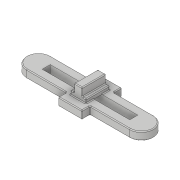
# Autodesk Inventor part: Slider1
Saved by Autodesk Inventor 2017 (Build 210142000, 142)
## iProperties
Created: 2016-07-28
Part Number: Slider1
Material: Generic
Document SubType Name: Modeling
Designer: Tutorial Books
Density: 1 g/cm^3
Appearance: Default
Author: Tutorial Books
Autodesk Inventor part; units mm, degrees
ref_plane "YZ Plane" through (0, 0, 0) normal (1, 0, 0) x (0, 1, 0)
ref_plane "XZ Plane" through (0, 0, 0) normal (0, 1, 0) x (-1, 0, 0)
ref_plane "XY Plane" through (0, 0, 0) normal (0, 0, 1) x (1, 0, 0)
sketch "Sketch1" plane through (0, 0, 0) normal (0, 1, 0) x (-1, 0, 0)
  arc A0 (64.897, -14.986) -> (64.897, 14.986) centre (64.897, 0) ccw
  arc A1 (-64.897, 14.986) -> (-64.897, -14.986) centre (-64.897, 0) ccw
  line L0 (64.897, 14.986) -> (14.986, 14.986)
  line L1 (14.986, 14.986) -> (14.986, 25.146)
  line L2 (14.986, 25.146) -> (-14.986, 25.146)
  line L3 (-14.986, 25.146) -> (-14.986, 14.986)
  line L4 (-14.986, 14.986) -> (-64.897, 14.986)
  line L5 (64.897, -14.986) -> (14.986, -14.986)
  line L6 (14.986, -14.986) -> (14.986, -25.146)
  line L7 (14.986, -25.146) -> (-14.986, -25.146)
  line L8 (-14.986, -25.146) -> (-14.986, -14.986)
  line L9 (-14.986, -14.986) -> (-64.897, -14.986)
  line L10 (0, 0) -> (0, -36.9179) construction
  line L11 (0, 0) -> (35.3103, 0) construction
  line L12 (55.245, 5.08) -> (-55.245, 5.08)
  line L13 (-55.245, 5.08) -> (-55.245, -5.08)
  line L14 (-55.245, -5.08) -> (55.245, -5.08)
  line L15 (55.245, -5.08) -> (55.245, 5.08)
  line L16 (55.245, 5.08) -> (-55.245, -5.08) construction
  line L17 (-55.245, 5.08) -> (55.245, -5.08) construction
  dimension "d0" = 129.794
  dimension "d1" = 14.986
  dimension "d2" = 29.972
  dimension "d3" = 110.49
  dimension "d4" = 10.16
  dimension "d5" = 10.16
  constraints: 36 end point, 6 horizontal, 6 point on line, 5 perpendicular, 4 point on circle, 3 tangent, 2 centre point, 2 midpoint, 2 parallel, 1 vertical, 4 other
  measures "d0" distance of A1.centre A0.centre
  measures "d1" radius of A0
  measures "d2" distance of L1.end L2.end
  measures "d3" distance of L13.end L14.end
  measures "d4" distance of L12.end L13.end
  measures "d5" distance of L0.end L1.end
extrude "Extrusion1" add sketch "Sketch1" along normal blind 10.16
sketch "Sketch2" plane through (0, 0, 0) normal (0, 0, 1) x (1, 0, 0)
  line L0 (-9.906, 10.16) -> (9.906, 10.16)
  line L1 (-14.986, 10.16) -> (14.986, 10.16) projected
  line L2 (9.906, 10.16) -> (9.906, 14.986)
  line L3 (9.906, 14.986) -> (5.08, 14.986)
  line L4 (5.08, 14.986) -> (5.08, 25.146)
  line L5 (5.08, 25.146) -> (-5.08, 25.146)
  line L6 (-5.08, 25.146) -> (-5.08, 14.986)
  line L7 (-5.08, 14.986) -> (-9.906, 14.986)
  line L8 (-9.906, 14.986) -> (-9.906, 10.16)
  line L9 (0, 0) -> (0, 16.6133) construction
  dimension "d8" = 19.812
  dimension "d9" = 10.16
  dimension "d10" = 10.16
  dimension "d11" = 4.826
  dimension "d12" = 5.08
  constraints: 18 end point, 5 perpendicular, 3 point on line, 2 vertical, 1 collinear
  measures "d8" distance between parallel lines of L8 L2
  measures "d9" distance of L3.end L4.end
  measures "d10" distance of L4.end L5.end
  measures "d11" distance of L0.end L2.end
  measures "d12" distance between parallel lines of L6 L9
extrude "Extrusion2" add sketch "Sketch2" along normal mid plane 29.972
fillet "Fillet1" radius 1.016 8 edges at (14.986, 5.08, 14.986) (14.986, 5.08, 25.146) (-14.986, 5.08, 25.146) (-14.986, 5.08, 14.986) (-14.986, 5.08, -14.986) (-14.986, 5.08, -25.146) (14.986, 5.08, -25.146) (14.986, 5.08, -14.986)
fillet "Fillet2" radius 1.016 40 edges at (79.883, 10.16, 0) (40.4495, 10.16, -14.986) (15.2836, 10.16, -15.2836) (14.986, 10.16, -20.066) (14.6884, 10.16, -24.8484) (0, 10.16, -25.146) (-14.6884, 10.16, -24.8484) (-14.986, 10.16, -20.066) (-15.2836, 10.16, -15.2836) (-40.4495, 10.16, -14.986) (-79.883, 10.16, 0) (-40.4495, 10.16, 14.986) (-15.2836, 10.16, 15.2836) (-14.986, 10.16, 20.066) (-14.6884, 10.16, 24.8484) (0, 10.16, 25.146) (14.6884, 10.16, 24.8484) (14.986, 10.16, 20.066) (15.2836, 10.16, 15.2836) (40.4495, 10.16, 14.986) (15.2836, 0, 15.2836) (14.986, 0, 20.066) (14.6884, 0, 24.8484) (0, 0, 25.146) (-14.6884, 0, 24.8484) (-14.986, 0, 20.066) (-15.2836, 0, 15.2836) (-40.4495, 0, 14.986) (-79.883, 0, 0) (-40.4495, 0, -14.986) (-15.2836, 0, -15.2836) (-14.986, 0, -20.066) (-14.6884, 0, -24.8484) (0, 0, -25.146) (14.6884, 0, -24.8484) (14.986, 0, -20.066) (15.2836, 0, -15.2836) (40.4495, 0, -14.986) (79.883, 0, 0) (40.4495, 0, 14.986)
fillet "Fillet3" radius 1.016 4 edges at (9.906, 12.573, 14.986) (-9.906, 12.573, 14.986) (9.906, 12.573, -14.986) (-9.906, 12.573, -14.986)
fillet "Fillet4" radius 1.016 10 edges at (-9.6084, 10.16, 14.6884) (-9.906, 10.16, 9.525) (9.6084, 10.16, 14.6884) (9.906, 10.16, 9.525) (0, 10.16, 14.986) (9.6084, 10.16, -14.6884) (0, 10.16, -14.986) (-9.6084, 10.16, -14.6884) (-9.906, 10.16, -9.525) (9.906, 10.16, -9.525)
fillet "Fillet5" radius 1.016 2 edges at (5.08, 14.986, 0) (-5.08, 14.986, 0)
fillet "Fillet6" radius 1.016 18 edges at (9.906, 14.986, 0) (9.6084, 14.986, 14.6884) (7.493, 14.986, 14.986) (5.3776, 15.2836, 14.986) (5.08, 20.574, 14.986) (7.493, 14.986, -14.986) (5.3776, 15.2836, -14.986) (5.08, 20.574, -14.986) (9.6084, 14.986, -14.6884) (-5.3776, 15.2836, 14.986) (-7.493, 14.986, 14.986) (-9.6084, 14.986, 14.6884) (-9.906, 14.986, 0) (-9.6084, 14.986, -14.6884) (-7.493, 14.986, -14.986) (-5.3776, 15.2836, -14.986) (-5.08, 20.574, -14.986) (-5.08, 20.574, 14.986)
fillet "Fillet7" radius 1.016 8 edges at (4.7824, 25.146, 14.6884) (0, 25.146, 14.986) (-4.7824, 25.146, 14.6884) (-5.08, 25.146, 0) (-4.7824, 25.146, -14.6884) (0, 25.146, -14.986) (4.7824, 25.146, -14.6884) (5.08, 25.146, 0)
body "Solid1"
